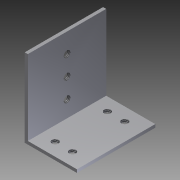
# Autodesk Inventor part: curveBracket
Saved by Autodesk Inventor 2011 SP1 (Build 150282100, 282)
## iProperties
Created: 2013-01-18
Part Number: curveBracket
Document SubType Name: Modeling
Designer: wes
Density: 1 g/cm^3
Author: wes
Autodesk Inventor part; units mm, degrees
ref_plane "YZ Plane" through (0, 0, 0) normal (1, 0, 0) x (0, 1, 0)
ref_plane "XZ Plane" through (0, 0, 0) normal (0, 1, 0) x (-1, 0, 0)
ref_plane "XY Plane" through (0, 0, 0) normal (0, 0, 1) x (1, 0, 0)
sketch "Sketch1" plane through (0, 0, 0) normal (0, 0, 1) x (1, 0, 0)
  line L0 (-30.7726, 64.3138) -> (-30.7726, -11.8862)
  line L1 (-30.7726, -11.8862) -> (20.0274, -11.8862)
  line L2 (20.0274, -11.8862) -> (20.0274, -8.8382)
  line L3 (20.0274, -8.8382) -> (-27.7246, -8.8382)
  line L4 (-27.7246, -8.8382) -> (-27.7246, 64.3138)
  line L5 (-27.7246, 64.3138) -> (-30.7726, 64.3138)
  point P0 (0, 0)
  dimension "d0" = 3.048
  dimension "d1" = 3.048
  dimension "d2" = 76.2
  dimension "d3" = 50.8
  constraints: 12 end point, 4 parallel, 1 perpendicular, 1 vertical
  measures "d0" distance of L4.end L0.start
  measures "d1" distance of L1.end L2.end
  measures "d2" distance of L0.start L0.end
  measures "d3" distance of L0.end L1.end
extrude "Extrusion1" add sketch "Sketch1" along normal blind 76.2
sketch "Sketch2" plane through (-30.7726, -11.8862, 0) normal (-1, 0, 0) x (0, 0, 1)
  line L0 (0, 76.2) -> (0, 0) projected
  line L1 (0, 0) -> (76.2, 0) projected
  point P0 (0, 11.8862)
  point P1 (38.1, 57.15)
  point P2 (38.1, 38.1)
  point P3 (38.1, 19.05)
  dimension "d6" = 19.05
  dimension "d7" = 38.1
  dimension "d8" = 57.15
  dimension "d9" = 38.1
  dimension "d10" = 38.1
  dimension "d11" = 38.1
  measures "d6" distance from line of L1 point (38.1, 19.05)
  measures "d7" distance from line of point (38.1, 38.1) L1
  measures "d8" distance from line of point (38.1, 57.15) L1
  measures "d9" distance from line of L0 point (38.1, 57.15)
  measures "d10" distance from line of L0 point (38.1, 38.1)
  measures "d11" distance from line of L0 point (38.1, 19.05)
hole "Hole1" at (-30.7726, 45.2638, 38.1) at (-30.7726, 26.2138, 38.1) at (-30.7726, 7.1638, 38.1) direction (1, 0, 0) diameter 6.35 depth 25.4 tip angle 118
thread "Thread1" size "1/4-20 UNC" class "2B" standard "ANSI Unified Screw Threads" full length
thread "Thread2" size "1/4-20 UNC" class "2B" standard "ANSI Unified Screw Threads" full length
thread "Thread3" size "1/4-20 UNC" class "2B" standard "ANSI Unified Screw Threads" full length
sketch "Sketch3" plane through (-27.7246, -8.8382, 0) normal (0, 1, 0) x (1, 0, 0)
  line L0 (0, -76.2) -> (47.752, -76.2) projected
  line L1 (47.752, 0) -> (47.752, -76.2) projected
  line L2 (47.752, 0) -> (0, 0) projected
  point P0 (27.7246, 0)
  point P1 (13.8853, -63.5)
  point P2 (13.8853, -12.7)
  point P3 (30.8187, -12.7)
  point P4 (30.8187, -63.5)
  dimension "d30" = 12.7
  dimension "d31" = 12.7
  dimension "d32" = 12.7
  dimension "d33" = 12.7
  dimension "d34" = 16.9333
  dimension "d35" = 33.8667
  dimension "d36" = 16.9333
  dimension "d37" = 33.8667
  measures "d30" distance from line of L2 point (30.819, -12.7)
  measures "d31" distance from line of point (13.885, -12.7) L2
  measures "d32" distance from line of L0 point (13.885, -63.5)
  measures "d33" distance from line of L0 point (30.819, -63.5)
  measures "d34" distance from line of L1 point (30.819, -12.7)
  measures "d35" distance from line of point (13.885, -12.7) L1
  measures "d36" distance from line of L1 point (30.819, -63.5)
  measures "d37" distance from line of L1 point (13.885, -63.5)
hole "Hole2" at (-13.8392, -8.8382, 63.5) at (-13.8392, -8.8382, 12.7) at (3.0941, -8.8382, 12.7) at (3.0941, -8.8382, 63.5) direction (0, -1, 0) diameter 6.35 depth 25.4 tip angle 118
thread "Thread4" size "1/4-20 UNC" class "2B" standard "ANSI Unified Screw Threads" full length
thread "Thread5" size "1/4-20 UNC" class "2B" standard "ANSI Unified Screw Threads" full length
thread "Thread6" size "1/4-20 UNC" class "2B" standard "ANSI Unified Screw Threads" full length
thread "Thread7" size "1/4-20 UNC" class "2B" standard "ANSI Unified Screw Threads" full length
body "Solid1"
